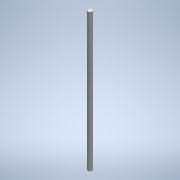
# Autodesk Inventor part: Lead Screw
Saved by Autodesk Inventor 2021 (Build 250183000, 183)
## iProperties
Created: 2021-08-04
Part Number: Lead Screw
Material: Generic
Document SubType Name: Modeling
Designer: techv
Density: 1 g/cm^3
Appearance: Default
Author: techv
Autodesk Inventor part; units mm, degrees
ref_plane "YZ Plane" through (0, 0, 0) normal (1, 0, 0) x (0, 1, 0)
ref_plane "XZ Plane" through (0, 0, 0) normal (0, 1, 0) x (-1, 0, 0)
ref_plane "XY Plane" through (0, 0, 0) normal (0, 0, 1) x (1, 0, 0)
sketch "Sketch1" plane through (0, 0, 0) normal (0, 1, 0) x (-1, 0, 0)
  circle A0 centre (0, 0) radius 1.5
  dimension "d0" = 3
  constraints: 1 centre point, 1 coincident
  measures "d0" diameter of A0
extrude "Extrusion1" add sketch "Sketch1" along normal blind 100
thread "Thread1" size "M3x0.5" class "6g" standard "ANSI Metric M Profile" full length
sketch "Sketch2" plane through (0, 0, 0) normal (0, -1, 0) x (1, 0, 0)
  circle A0 centre (0, 0) radius 1.5 projected
  line L0 (-1.3477, 0.6586) -> (1.3477, 0.6586)
  constraints: 2 end point, 2 point on circle, 1 horizontal
extrude "Extrusion2" add sketch "Sketch2" along normal blind 4 contours A0 L0 picked at (-0.2882, -0.1605)
body "Solid1"
